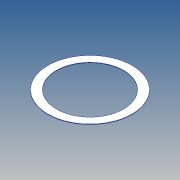
# Autodesk Inventor part: Zylinderbuchsenring_ra8846s
Saved by Autodesk Inventor 2021 (Build 250183000, 183)
## iProperties
Created: 2020-11-16
Part Number: Zylinderbuchsenring_ra8846s
Material: Aluminium 6061
Document SubType Name: Modeling
Designer: Ricardo A
Density: 2.7 g/cm^3
Appearance: Aluminium - flach
Description: Motor_Teil3_ring
Mass: 0.0233793 g
Surface Area: 1.83076 cm^2
Volume: 0.00865901 cm^3
Author: Ricardo A
Revision Number: Rev00
Autodesk Inventor part; units mm, degrees
ref_plane "YZ-Ebene" through (0, 0, 0) normal (1, 0, 0) x (0, 1, 0)
ref_plane "XZ-Ebene" through (0, 0, 0) normal (0, 1, 0) x (-1, 0, 0)
ref_plane "XY-Ebene" through (0, 0, 0) normal (0, 0, 1) x (1, 0, 0)
sketch "Skizze1" plane through (0, 0, 0) normal (0, 0, 1) x (1, 0, 0)
  line L0 (-12.25, 0) -> (12.25, 0) projected
  line L1 (0, -12.25) -> (0, 12.25) projected
  circle A0 centre (0, 0) radius 7
  circle A1 centre (0, 0) radius 8.75
  dimension "d0" = 14
  dimension "d1" = 17.5
  constraints: 2 centre point, 2 coincident
  measures "d0" diameter of A0
  measures "d1" diameter of A1
extrude "Extrusion1" add sketch "Skizze1" along normal blind 0.1 contours A0 L1 A1 L0 | L0 A1 L1 A0 | A0 L0 A1 L1 | L1 A1 L0 A0
